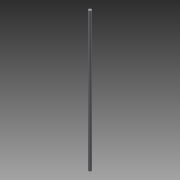
# Autodesk Inventor part: y axis 8mm rod
Saved by Autodesk Inventor 2013 SP2 (Build 170200200, 200)
## iProperties
Created: 2017-03-11
Part Number: y axis 8mm rod
Material: Generic
Document SubType Name: Modeling
Designer: Herman de Vries
Density: 1 g/cm^3
Mass: 19.1009 g
Surface Area: 96.5097 cm^2
Volume: 19.1009 cm^3
Author: Herman de Vries
Autodesk Inventor part; units mm, degrees
ref_plane "YZ Plane" through (0, 0, 0) normal (1, 0, 0) x (0, 1, 0)
ref_plane "XZ Plane" through (0, 0, 0) normal (0, 1, 0) x (-1, 0, 0)
ref_plane "XY Plane" through (0, 0, 0) normal (0, 0, 1) x (1, 0, 0)
sketch "Sketch1" plane through (0, 0, 0) normal (0, 0, 1) x (1, 0, 0)
  circle A0 centre (0, 0) radius 4
  dimension "d0" = 8
  constraints: 1 centre point, 1 coincident
  measures "d0" diameter of A0
extrude "Extrusion1" add sketch "Sketch1" along normal blind 380
body "Solid1"
